Autodesk Fusion 360 part; units mm, degrees
(part 21 of 25)
  arc A482 (48.133, 42.8879) -> (48.133, 42.9641) centre (48.133, 42.926) ccw
  arc A483 (48.26, 36.9951) -> (48.26, 36.9189) centre (48.26, 36.957) ccw
  line L257 (48.895, 41.021) -> (48.895, 42.799)
  arc A484 (43.307, 39.1541) -> (43.307, 39.0779) centre (43.307, 39.116) ccw
  line L258 (48.133, 40.894) -> (43.307, 40.894)
  arc A485 (43.2801, 39.0891) -> (43.3339, 39.1429) centre (43.307, 39.116) ccw
  arc A486 (43.2069, 39.2699) -> (43.1531, 39.2161) centre (43.18, 39.243) ccw
  arc A487 (48.641, 36.9189) -> (48.641, 36.9951) centre (48.641, 36.957) ccw
  arc A488 (48.133, 37.0459) -> (48.133, 37.1221) centre (48.133, 37.084) ccw
  arc A489 (48.9331, 41.021) -> (48.8569, 41.021) centre (48.895, 41.021) ccw
  line L259 (42.799, 43.053) -> (43.18, 43.053)
  arc A490 (48.2869, 43.0261) -> (48.2331, 43.0799) centre (48.26, 43.053) ccw
  arc A491 (48.641, 43.0149) -> (48.641, 43.0911) centre (48.641, 43.053) ccw
  arc A492 (28.5369, 41.021) -> (28.6131, 41.021) centre (28.575, 41.021) ccw
  line L260 (42.799, 40.767) -> (43.18, 40.767)
  line L261 (48.133, 42.926) -> (43.307, 42.926)
  arc A493 (48.26, 40.8051) -> (48.26, 40.7289) centre (48.26, 40.767) ccw
  arc A494 (48.641, 40.8051) -> (48.641, 40.7289) centre (48.641, 40.767) ccw
  arc A495 (48.1061, 42.9529) -> (48.1599, 42.8991) centre (48.133, 42.926) ccw
  arc A496 (48.641, 43.0911) -> (48.641, 43.0149) centre (48.641, 43.053) ccw
  arc A497 (42.5831, 42.799) -> (42.5069, 42.799) centre (42.545, 42.799) ccw
  arc A498 (42.799, 40.8051) -> (42.799, 40.7289) centre (42.799, 40.767) ccw
  arc A499 (43.307, 42.9641) -> (43.307, 42.8879) centre (43.307, 42.926) ccw
  arc A500 (43.18, 43.0149) -> (43.18, 43.0911) centre (43.18, 43.053) ccw
  arc A501 (48.133, 40.8559) -> (48.133, 40.9321) centre (48.133, 40.894) ccw
  arc A502 (48.26, 43.0911) -> (48.26, 43.0149) centre (48.26, 43.053) ccw
  line L262 (29.337, 42.926) -> (29.21, 43.053)
  line L263 (48.641, 43.053) -> (48.26, 43.053)
  arc A503 (29.3639, 40.8671) -> (29.3101, 40.9209) centre (29.337, 40.894) ccw
  arc A504 (43.3339, 40.8671) -> (43.2801, 40.9209) centre (43.307, 40.894) ccw
  arc A505 (29.1831, 40.7939) -> (29.2369, 40.7401) centre (29.21, 40.767) ccw
  arc A506 (34.29, 43.0911) -> (34.29, 43.0149) centre (34.29, 43.053) ccw
  arc A507 (28.829, 40.8051) -> (28.829, 40.7289) centre (28.829, 40.767) ccw
  arc A508 (42.799, 43.0911) -> (42.799, 43.0149) centre (42.799, 43.053) ccw
  arc A509 (48.2331, 40.7401) -> (48.2869, 40.7939) centre (48.26, 40.767) ccw
  line L264 (34.163, 40.894) -> (34.29, 40.767)
  arc A510 (42.799, 43.053) -> (42.545, 42.799) centre (42.799, 42.799) ccw
  arc A511 (42.5069, 41.021) -> (42.5831, 41.021) centre (42.545, 41.021) ccw
  arc A512 (42.799, 43.0149) -> (42.799, 43.0911) centre (42.799, 43.053) ccw
  line L265 (42.545, 41.6052) -> (42.545, 42.2148)
  line L266 (49.7586, 41.6052) -> (49.7586, 42.2148)
  line L267 (41.6814, 42.2148) -> (41.6814, 41.6052)
  arc A513 (43.2069, 43.0799) -> (43.1531, 43.0261) centre (43.18, 43.053) ccw
  line L268 (28.829, 43.053) -> (29.21, 43.053)
  arc A514 (29.3101, 42.8991) -> (29.3639, 42.9529) centre (29.337, 42.926) ccw
  arc A515 (43.1531, 40.7939) -> (43.2069, 40.7401) centre (43.18, 40.767) ccw
  arc A516 (34.671, 40.7289) -> (34.671, 40.8051) centre (34.671, 40.767) ccw
  line L269 (43.307, 42.926) -> (43.18, 43.053)
  line L270 (34.671, 40.767) -> (34.29, 40.767)
  arc A517 (48.9331, 42.799) -> (48.8569, 42.799) centre (48.895, 42.799) ccw
  arc A518 (42.545, 41.021) -> (42.799, 40.767) centre (42.799, 41.021) ccw
  arc A519 (34.163, 42.8879) -> (34.163, 42.9641) centre (34.163, 42.926) ccw
  arc A520 (34.671, 40.767) -> (34.925, 41.021) centre (34.671, 41.021) ccw
  line L271 (28.575, 41.021) -> (28.575, 42.799)
  arc A521 (48.8569, 41.021) -> (48.9331, 41.021) centre (48.895, 41.021) ccw
  arc A522 (48.641, 40.7289) -> (48.641, 40.8051) centre (48.641, 40.767) ccw
  arc A523 (34.163, 40.8559) -> (34.163, 40.9321) centre (34.163, 40.894) ccw
  line L272 (48.133, 40.894) -> (48.26, 40.767)
  line L273 (42.545, 42.2148) -> (41.6814, 42.2148)
  line L274 (49.7586, 42.2148) -> (48.895, 42.2148)
  arc A524 (34.9631, 41.021) -> (34.8869, 41.021) centre (34.925, 41.021) ccw
  arc A525 (34.671, 43.0149) -> (34.671, 43.0911) centre (34.671, 43.053) ccw
  arc A526 (42.5831, 41.021) -> (42.5069, 41.021) centre (42.545, 41.021) ccw
  arc A527 (34.8869, 42.799) -> (34.9631, 42.799) centre (34.925, 42.799) ccw
  arc A528 (28.575, 41.021) -> (28.829, 40.767) centre (28.829, 41.021) ccw
  arc A529 (48.641, 40.767) -> (48.895, 41.021) centre (48.641, 41.021) ccw
  line L275 (41.6814, 41.6052) -> (42.545, 41.6052)
  arc A530 (34.671, 43.0911) -> (34.671, 43.0149) centre (34.671, 43.053) ccw
  arc A531 (13.081, 16.4211) -> (13.081, 16.3449) centre (13.081, 16.383) ccw
  arc A532 (28.6131, 42.799) -> (28.5369, 42.799) centre (28.575, 42.799) ccw
  arc A533 (34.9631, 42.799) -> (34.8869, 42.799) centre (34.925, 42.799) ccw
  arc A534 (13.081, 16.3449) -> (13.081, 16.4211) centre (13.081, 16.383) ccw
  arc A535 (34.925, 42.799) -> (34.671, 43.053) centre (34.671, 42.799) ccw
  arc A536 (34.29, 40.8051) -> (34.29, 40.7289) centre (34.29, 40.767) ccw
  arc A537 (28.829, 43.053) -> (28.575, 42.799) centre (28.829, 42.799) ccw
  arc A538 (29.337, 42.9641) -> (29.337, 42.8879) centre (29.337, 42.926) ccw
  arc A539 (34.2631, 40.7401) -> (34.3169, 40.7939) centre (34.29, 40.767) ccw
  arc A540 (29.21, 43.0149) -> (29.21, 43.0911) centre (29.21, 43.053) ccw
  arc A541 (34.671, 40.8051) -> (34.671, 40.7289) centre (34.671, 40.767) ccw
  arc A542 (28.829, 43.0149) -> (28.829, 43.0911) centre (28.829, 43.053) ccw
  arc A543 (7.7739, 14.1971) -> (7.7201, 14.2509) centre (7.747, 14.224) ccw
  line L276 (13.081, 16.383) -> (12.7, 16.383)
  line L277 (28.829, 40.767) -> (29.21, 40.767)
  line L278 (27.7114, 42.2148) -> (27.7114, 41.6052)
  arc A544 (28.6131, 41.021) -> (28.5369, 41.021) centre (28.575, 41.021) ccw
  line L279 (34.925, 41.021) -> (34.925, 42.799)
  arc A545 (34.3169, 43.0261) -> (34.2631, 43.0799) centre (34.29, 43.053) ccw
  arc A546 (12.5999, 14.2509) -> (12.5461, 14.1971) centre (12.573, 14.224) ccw
  arc A547 (7.6469, 16.4099) -> (7.5931, 16.3561) centre (7.62, 16.383) ccw
  arc A548 (29.21, 40.7289) -> (29.21, 40.8051) centre (29.21, 40.767) ccw
  line L280 (34.925, 41.6052) -> (35.7886, 41.6052)
  arc A549 (12.573, 14.1859) -> (12.573, 14.2621) centre (12.573, 14.224) ccw
  line L281 (28.575, 41.6052) -> (28.575, 42.2148)
  line L282 (35.7886, 42.2148) -> (34.925, 42.2148)
  arc A550 (28.829, 43.0911) -> (28.829, 43.0149) centre (28.829, 43.053) ccw
  line L283 (27.7114, 41.6052) -> (28.575, 41.6052)
  arc A551 (13.081, 14.097) -> (13.335, 14.351) centre (13.081, 14.351) ccw
  line L284 (7.747, 16.256) -> (12.573, 16.256)
  arc A552 (7.239, 16.383) -> (6.985, 16.129) centre (7.239, 16.129) ccw
  arc A553 (12.7, 14.1351) -> (12.7, 14.0589) centre (12.7, 14.097) ccw
  line L285 (12.573, 16.256) -> (12.7, 16.383)
  line L286 (13.335, 16.129) -> (13.335, 14.351)
  line L287 (29.337, 40.894) -> (29.21, 40.767)
  arc A554 (34.1899, 40.9209) -> (34.1361, 40.8671) centre (34.163, 40.894) ccw
  arc A555 (28.829, 40.7289) -> (28.829, 40.8051) centre (28.829, 40.767) ccw
  arc A556 (13.2969, 14.351) -> (13.3731, 14.351) centre (13.335, 14.351) ccw
  line L288 (35.7886, 41.6052) -> (35.7886, 42.2148)
  line L289 (34.671, 43.053) -> (34.29, 43.053)
  arc A557 (6.9469, 16.129) -> (7.0231, 16.129) centre (6.985, 16.129) ccw
  arc A558 (12.573, 16.2179) -> (12.573, 16.2941) centre (12.573, 16.256) ccw
  arc A559 (7.0231, 14.351) -> (6.9469, 14.351) centre (6.985, 14.351) ccw
  arc A560 (29.2369, 43.0799) -> (29.1831, 43.0261) centre (29.21, 43.053) ccw
  line L290 (13.081, 14.097) -> (12.7, 14.097)
  arc A561 (7.747, 16.2941) -> (7.747, 16.2179) centre (7.747, 16.256) ccw
  arc A562 (7.239, 14.0589) -> (7.239, 14.1351) centre (7.239, 14.097) ccw
  arc A563 (34.8869, 41.021) -> (34.9631, 41.021) centre (34.925, 41.021) ccw
  line L291 (7.747, 14.224) -> (7.62, 14.097)
  line L292 (34.925, 42.2148) -> (34.925, 41.6052)
  arc A564 (13.335, 16.129) -> (13.081, 16.383) centre (13.081, 16.129) ccw
  arc A565 (28.5369, 42.799) -> (28.6131, 42.799) centre (28.575, 42.799) ccw
  line L293 (34.163, 42.926) -> (34.29, 43.053)
  line L294 (12.573, 14.224) -> (12.7, 14.097)
  line L295 (34.163, 40.894) -> (29.337, 40.894)
  arc A566 (12.6731, 14.0701) -> (12.7269, 14.1239) centre (12.7, 14.097) ccw
  line L296 (34.163, 42.926) -> (29.337, 42.926)
  line L297 (28.575, 42.2148) -> (27.7114, 42.2148)
  line L298 (7.747, 16.256) -> (7.62, 16.383)
  arc A567 (29.337, 40.9321) -> (29.337, 40.8559) centre (29.337, 40.894) ccw
  arc A568 (34.1361, 42.9529) -> (34.1899, 42.8991) centre (34.163, 42.926) ccw
  arc A569 (13.3731, 16.129) -> (13.2969, 16.129) centre (13.335, 16.129) ccw
  arc A570 (13.081, 14.1351) -> (13.081, 14.0589) centre (13.081, 14.097) ccw
  arc A571 (12.7, 16.4211) -> (12.7, 16.3449) centre (12.7, 16.383) ccw
  line L299 (6.985, 15.5448) -> (6.1214, 15.5448)
  line L300 (7.747, 14.224) -> (12.573, 14.224)
  arc A572 (12.5461, 16.2829) -> (12.5999, 16.2291) centre (12.573, 16.256) ccw
  arc A573 (13.3731, 14.351) -> (13.2969, 14.351) centre (13.335, 14.351) ccw
  arc A574 (7.239, 16.3449) -> (7.239, 16.4211) centre (7.239, 16.383) ccw
  arc A575 (7.239, 14.1351) -> (7.239, 14.0589) centre (7.239, 14.097) ccw
  line L301 (6.1214, 14.9352) -> (6.985, 14.9352)
  arc A576 (7.62, 16.3449) -> (7.62, 16.4211) centre (7.62, 16.383) ccw
  arc A577 (7.62, 14.0589) -> (7.62, 14.1351) centre (7.62, 14.097) ccw
  arc A578 (12.7269, 16.3561) -> (12.6731, 16.4099) centre (12.7, 16.383) ccw
  arc A579 (7.747, 14.2621) -> (7.747, 14.1859) centre (7.747, 14.224) ccw
  arc A580 (6.9469, 14.351) -> (7.0231, 14.351) centre (6.985, 14.351) ccw
  arc A581 (13.2969, 16.129) -> (13.3731, 16.129) centre (13.335, 16.129) ccw
  arc A582 (13.081, 14.0589) -> (13.081, 14.1351) centre (13.081, 14.097) ccw
  arc A583 (6.985, 14.351) -> (7.239, 14.097) centre (7.239, 14.351) ccw
  line L302 (7.239, 14.097) -> (7.62, 14.097)
  arc A584 (7.5931, 14.1239) -> (7.6469, 14.0701) centre (7.62, 14.097) ccw
  arc A585 (7.7201, 16.2291) -> (7.7739, 16.2829) centre (7.747, 16.256) ccw
  line L303 (13.335, 14.9352) -> (14.1986, 14.9352)
  arc A586 (21.4559, 38.2265) -> (21.971, 38.545) centre (20.3211, 40.6376) ccw
  arc A587 (19.1706, 38.1983) -> (19.1976, 38.2557) centre (19.1841, 38.227) ccw
  arc A588 (80.4672, 18.034) -> (80.5688, 18.034) centre (80.518, 18.034) ccw
  arc A589 (5.207, 29.1465) -> (5.207, 29.2735) centre (5.207, 29.21) ccw
  arc A590 (80.5688, 20.048) -> (80.4672, 20.048) centre (80.518, 20.048) ccw
  line L304 (74.4499, 6.1715) -> (74.4499, 4.1275)
  arc A591 (7.62, 26.67) -> (7.62, 24.13) centre (7.62, 25.4) ccw
  arc A592 (4.5085, 28.575) -> (4.6355, 28.575) centre (4.572, 28.575) ccw
  arc A593 (7.239, 16.4211) -> (7.239, 16.3449) centre (7.239, 16.383) ccw
  arc A594 (80.4951, 4.1275) -> (80.5967, 4.1275) centre (80.5459, 4.1275) ccw
  arc A595 (74.3991, 4.1275) -> (74.5007, 4.1275) centre (74.4499, 4.1275) ccw
  line L305 (13.335, 15.5448) -> (13.335, 14.9352)
  arc A596 (75.311, 22.1488) -> (75.311, 22.0472) centre (75.311, 22.098) ccw
  arc A597 (7.62, 18.415) -> (7.62, 32.385) centre (7.62, 25.4) ccw
  line L306 (79.629, 22.098) -> (75.311, 22.098)
  arc A598 (79.629, 15.9512) -> (79.629, 16.0528) centre (79.629, 16.002) ccw
  line L307 (75.3389, 2.0955) -> (79.6569, 2.0955)
  line L308 (80.518, 20.048) -> (80.518, 18.034)
  arc A599 (4.6355, 29.845) -> (4.5085, 29.845) centre (4.572, 29.845) ccw
  line L309 (21.971, 38.545) -> (21.971, 42.735)
  line L310 (80.5459, 6.1415) -> (80.5459, 4.1275)
  arc A600 (79.6569, 8.1407) -> (79.6569, 8.2423) centre (79.6569, 8.1915) ccw
  arc A601 (75.3389, 2.1463) -> (75.3389, 2.0447) centre (75.3389, 2.0955) ccw
  arc A602 (77.47, 17.272) -> (77.47, 20.828) centre (77.47, 19.05) ccw
  arc A603 (77.47, 20.828) -> (77.47, 17.272) centre (77.47, 19.05) ccw
  line L311 (6.985, 14.9352) -> (6.985, 15.5448)
  arc A604 (77.4979, 6.9215) -> (77.4979, 3.3655) centre (77.4979, 5.1435) ccw
  arc A605 (4.572, 30.48) -> (4.572, 27.94) centre (4.572, 29.21) ccw
  arc A606 (7.62, 24.13) -> (7.62, 26.67) centre (7.62, 25.4) ccw
  arc A607 (77.4979, 3.3655) -> (77.4979, 6.9215) centre (77.4979, 5.1435) ccw
  arc A608 (75.311, 16.0528) -> (75.311, 15.9512) centre (75.311, 16.002) ccw
  line L312 (14.1986, 15.5448) -> (13.335, 15.5448)
  arc A609 (79.6569, 2.0447) -> (79.6569, 2.1463) centre (79.6569, 2.0955) ccw
  arc A610 (74.4728, 20.078) -> (74.3712, 20.078) centre (74.422, 20.078) ccw
  arc A611 (21.9513, 42.7101) -> (21.9907, 42.7599) centre (21.971, 42.735) ccw
  arc A612 (79.629, 22.0472) -> (79.629, 22.1488) centre (79.629, 22.098) ccw
  arc A613 (4.572, 27.94) -> (4.572, 30.48) centre (4.572, 29.21) ccw
  line L313 (4.572, 28.575) -> (4.572, 29.845)
  arc A614 (20.4788, 42.044) -> (20.4153, 42.044) centre (20.4471, 42.044) ccw
  line L314 (14.1986, 14.9352) -> (14.1986, 15.5448)
  line L315 (6.985, 16.129) -> (6.985, 14.351)
  arc A615 (75.3389, 8.2423) -> (75.3389, 8.1407) centre (75.3389, 8.1915) ccw
  arc A616 (7.0231, 16.129) -> (6.9469, 16.129) centre (6.985, 16.129) ccw
  line L316 (6.1214, 15.5448) -> (6.1214, 14.9352)
  line L317 (7.239, 16.383) -> (7.62, 16.383)
  arc A617 (80.5967, 6.1415) -> (80.4951, 6.1415) centre (80.5459, 6.1415) ccw
  line L318 (75.311, 16.002) -> (79.629, 16.002)
  arc A618 (74.3712, 18.034) -> (74.4728, 18.034) centre (74.422, 18.034) ccw
  line L319 (3.937, 29.21) -> (5.207, 29.21)
  arc A619 (7.62, 32.385) -> (7.62, 18.415) centre (7.62, 25.4) ccw
  arc A620 (3.937, 29.2735) -> (3.937, 29.1465) centre (3.937, 29.21) ccw
  arc A621 (74.5007, 6.1715) -> (74.3991, 6.1715) centre (74.4499, 6.1715) ccw
  line L320 (79.6569, 8.1915) -> (75.3389, 8.1915)
  line L321 (74.422, 20.078) -> (74.422, 18.034)
  arc A622 (21.445, 43.0936) -> (21.4186, 43.0358) centre (21.4318, 43.0647) ccw
  arc A623 (20.4788, 39.504) -> (20.4153, 39.504) centre (20.4471, 39.504) ccw
  arc A624 (20.4153, 39.236) -> (20.4788, 39.236) centre (20.4471, 39.236) ccw
  arc A625 (20.4153, 41.776) -> (20.4788, 41.776) centre (20.4471, 41.776) ccw
  arc A626 (22.0027, 42.735) -> (21.9393, 42.735) centre (21.971, 42.735) ccw
  line L322 (20.447, 42.044) -> (20.447, 41.776)
  arc A627 (21.9393, 38.545) -> (22.0027, 38.545) centre (21.971, 38.545) ccw
  arc A628 (19.1841, 43.053) -> (19.1841, 38.227) centre (20.3201, 40.64) ccw
  arc A629 (21.9907, 38.5201) -> (21.9513, 38.5699) centre (21.971, 38.545) ccw
  arc A630 (21.971, 42.735) -> (21.4318, 43.0647) centre (20.321, 40.6423) ccw
  arc A631 (21.4424, 38.2552) -> (21.4694, 38.1978) centre (21.4559, 38.2265) ccw
  arc A632 (19.1976, 43.0243) -> (19.1706, 43.0817) centre (19.1841, 43.053) ccw
  line L323 (20.447, 39.504) -> (20.447, 39.236)
  line L324 (75.311, 22.098) -> (74.422, 22.098)
  line L325 (74.422, 22.098) -> (74.422, 20.078)
  line L326 (74.422, 18.034) -> (74.422, 16.002)
  line L327 (74.422, 16.002) -> (75.311, 16.002)
  line L328 (79.629, 16.002) -> (80.518, 16.002)
  line L329 (80.518, 16.002) -> (80.518, 18.034)
  line L330 (79.629, 22.098) -> (80.518, 22.098)
  line L331 (80.518, 22.098) -> (80.518, 20.048)
  line L332 (75.3389, 8.1915) -> (74.4499, 8.1915)
  line L333 (74.4499, 8.1915) -> (74.4499, 6.1715)
  line L334 (74.4499, 4.1275) -> (74.4499, 2.0955)
  line L335 (74.4499, 2.0955) -> (75.3389, 2.0955)
  line L336 (79.6569, 2.0955) -> (80.5459, 2.0955)
  line L337 (80.5459, 2.0955) -> (80.5459, 4.1275)
  line L338 (79.6569, 8.1915) -> (80.5459, 8.1915)
  line L339 (80.5459, 8.1915) -> (80.5459, 6.1415)
  arc A633 (21.4318, 43.0647) -> (19.1841, 43.053) centre (20.3205, 40.6413) ccw
  arc A634 (19.1841, 38.227) -> (21.4559, 38.2265) centre (20.3205, 40.641) ccw
  arc A635 (14.8844, 6.2992) -> (13.0344, 6.283) centre (13.97, 5.0798) ccw
  arc A636 (13.0344, 3.877) -> (14.8558, 3.8399) centre (13.97, 5.0802) ccw
  arc A637 (5.9817, 6.2865) -> (4.1317, 6.2703) centre (5.0673, 5.0671) ccw
  arc A638 (4.1317, 3.8643) -> (5.9531, 3.8272) centre (5.0673, 5.0675) ccw
  constraint coincident A596.centre L306.end
  constraint perpendicular L321 L324
  constraint coincident A610.centre L321.start
  constraint perpendicular L324 L325
  constraint coincident A618.centre L321.end
  constraint perpendicular L318 L326
  constraint coincident A608.centre L318.start
  constraint perpendicular L326 L327
  constraint coincident A598.centre L318.end
  constraint perpendicular L308 L328
  constraint coincident A588.centre L308.end
  constraint perpendicular L328 L329
  constraint coincident L306.start A612.centre
  constraint perpendicular L308 L330
  constraint coincident A590.centre L308.start
  constraint perpendicular L330 L331
  constraint coincident A615.centre L320.end
  constraint perpendicular L304 L332
  constraint coincident L304.start A621.centre
  constraint perpendicular L332 L333
  constraint coincident L304.end A595.centre
  constraint perpendicular L307 L334
  constraint coincident L307.start A601.centre
  constraint perpendicular L334 L335
  constraint coincident L307.end A609.centre
  constraint perpendicular L310 L336
  constraint coincident A594.centre L310.end
  constraint perpendicular L336 L337
  constraint coincident A600.centre L320.start
  constraint perpendicular L310 L338
  constraint coincident L310.start A617.centre
  constraint perpendicular L320 L339
  constraint coincident A622.centre A630.end
  constraint tangent A630 A633
  constraint tangent A628 A634
  constraint tangent A222 A635
  constraint tangent A238 A636
  constraint tangent A171 A638
  constraint tangent A242 A637
sketch "Through Holes" plane through (0, 0, 0) normal (0, 0, 1) x (1, 0, 0)
  line L0 (72.5558, 49.13) -> (72.2242, 49.13)
  line L1 (72.2242, 49.13) -> (71.99, 49.3642)
  line L2 (72.7901, 49.6958) -> (72.7901, 49.3642)
  line L3 (72.2242, 49.9301) -> (72.5558, 49.9301)
  line L4 (74.53, 49.6958) -> (74.7642, 49.9301)
  line L5 (71.99, 49.3642) -> (71.99, 49.6958)
  arc A0 (68.1101, 6.35) -> (69.0499, 6.35) centre (68.58, 6.35) ccw
  line L6 (74.7642, 49.13) -> (74.53, 49.3642)
  line L7 (75.0958, 49.13) -> (74.7642, 49.13)
  line L8 (71.99, 49.6958) -> (72.2242, 49.9301)
  line L9 (74.7642, 49.9301) -> (75.0958, 49.9301)
  line L10 (72.2242, 49.9301) -> (72.5558, 49.9301)
  line L11 (74.53, 49.3642) -> (74.53, 49.6958)
  line L12 (75.0958, 49.13) -> (74.7642, 49.13)
  line L13 (75.3301, 49.3642) -> (75.0958, 49.13)
  line L14 (72.5558, 49.9301) -> (72.7901, 49.6958)
  arc A1 (66.5099, 6.35) -> (65.5701, 6.35) centre (66.04, 6.35) ccw
  line L15 (72.7901, 49.3642) -> (72.5558, 49.13)
  line L16 (74.7642, 49.9301) -> (75.0958, 49.9301)
  line L17 (74.7642, 49.13) -> (74.53, 49.3642)
  line L18 (72.7901, 49.3642) -> (72.5558, 49.13)
  line L19 (72.2242, 49.13) -> (71.99, 49.3642)
  line L20 (71.99, 49.3642) -> (71.99, 49.6958)
  line L21 (74.53, 49.6958) -> (74.7642, 49.9301)
  line L22 (71.99, 49.3642) -> (71.99, 49.6958)
  line L23 (75.3301, 49.3642) -> (75.0958, 49.13)
  line L24 (53.1558, 17.3355) -> (52.8955, 17.5958)
  line L25 (53.7845, 17.5958) -> (53.5242, 17.3355)
  arc A2 (50.8, 18.2245) -> (50.8, 17.3355) centre (50.8, 17.78) ccw
  line L26 (53.5242, 17.3355) -> (53.1558, 17.3355)
  line L27 (74.53, 49.3642) -> (74.53, 49.6958)
  arc A3 (50.8, 17.3355) -> (50.8, 18.2245) centre (50.8, 17.78) ccw
  line L28 (53.1558, 18.2245) -> (53.5242, 18.2245)
  arc A4 (50.8, 18.2245) -> (50.8, 17.3355) centre (50.8, 17.78) ccw
  line L29 (72.7901, 49.6958) -> (72.7901, 49.3642)
  line L30 (75.3301, 49.6958) -> (75.3301, 49.3642)
  line L31 (53.5242, 18.2245) -> (53.7845, 17.9642)
  line L32 (52.8955, 17.5958) -> (52.8955, 17.9642)
  line L33 (52.8955, 17.9642) -> (53.1558, 18.2245)
  arc A5 (65.5701, 6.35) -> (66.5099, 6.35) centre (66.04, 6.35) ccw
  line L34 (74.53, 49.3642) -> (74.53, 49.6958)
  arc A6 (69.0499, 6.35) -> (68.1101, 6.35) centre (68.58, 6.35) ccw
  line L35 (74.53, 49.3642) -> (74.53, 49.6958)
  line L36 (72.5558, 49.13) -> (72.2242, 49.13)
  line L37 (75.3301, 49.6958) -> (75.3301, 49.3642)
  line L38 (71.99, 49.6958) -> (72.2242, 49.9301)
  line L39 (72.5558, 49.9301) -> (72.7901, 49.6958)
  line L40 (52.8955, 17.5958) -> (52.8955, 17.9642)
  line L41 (75.0958, 49.9301) -> (75.3301, 49.6958)
  line L42 (75.0958, 49.9301) -> (75.3301, 49.6958)
  line L43 (71.99, 49.3642) -> (71.99, 49.6958)
  arc A7 (61.4299, 6.35) -> (60.4901, 6.35) centre (60.96, 6.35) ccw
  arc A8 (40.1701, 6.35) -> (41.1099, 6.35) centre (40.64, 6.35) ccw
  arc A9 (57.9501, 6.35) -> (58.8899, 6.35) centre (58.42, 6.35) ccw
  arc A10 (14.3891, 33.909) -> (13.5509, 33.909) centre (13.97, 33.909) ccw
  arc A11 (4.318, 50.3555) -> (4.318, 53.5305) centre (4.318, 51.943) ccw
  arc A12 (14.3891, 44.069) -> (13.5509, 44.069) centre (13.97, 44.069) ccw
  arc A13 (50.8, 17.3355) -> (50.8, 18.2245) centre (50.8, 17.78) ccw
  arc A14 (33.4899, 6.35) -> (32.5501, 6.35) centre (33.02, 6.35) ccw
  arc A15 (50.3301, 6.35) -> (51.2699, 6.35) centre (50.8, 6.35) ccw
  arc A16 (41.1099, 6.35) -> (40.1701, 6.35) centre (40.64, 6.35) ccw
  arc A17 (45.2501, 6.35) -> (46.1899, 6.35) centre (45.72, 6.35) ccw
  arc A18 (61.4299, 6.35) -> (60.4901, 6.35) centre (60.96, 6.35) ccw
  arc A19 (4.318, 50.3555) -> (4.318, 53.5305) centre (4.318, 51.943) ccw
  arc A20 (45.2501, 6.35) -> (46.1899, 6.35) centre (45.72, 6.35) ccw
  arc A21 (40.1701, 6.35) -> (41.1099, 6.35) centre (40.64, 6.35) ccw
  arc A22 (63.9699, 6.35) -> (63.0301, 6.35) centre (63.5, 6.35) ccw
  arc A23 (66.5099, 6.35) -> (65.5701, 6.35) centre (66.04, 6.35) ccw
  arc A24 (13.5509, 33.909) -> (14.3891, 33.909) centre (13.97, 33.909) ccw
  arc A25 (14.3891, 44.069) -> (13.5509, 44.069) centre (13.97, 44.069) ccw
  arc A26 (80.645, 50.3555) -> (80.645, 53.5305) centre (80.645, 51.943) ccw
  arc A27 (58.8899, 6.35) -> (57.9501, 6.35) centre (58.42, 6.35) ccw
  arc A28 (68.1101, 6.35) -> (69.0499, 6.35) centre (68.58, 6.35) ccw
  arc A29 (37.6301, 6.35) -> (38.5699, 6.35) centre (38.1, 6.35) ccw
  arc A30 (35.0901, 6.35) -> (36.0299, 6.35) centre (35.56, 6.35) ccw
  line L44 (53.1558, 18.2245) -> (53.5242, 18.2245)
  arc A31 (14.3891, 33.909) -> (13.5509, 33.909) centre (13.97, 33.909) ccw
  arc A32 (13.5509, 44.069) -> (14.3891, 44.069) centre (13.97, 44.069) ccw
  arc A33 (32.5501, 6.35) -> (33.4899, 6.35) centre (33.02, 6.35) ccw
  arc A34 (50.3301, 6.35) -> (51.2699, 6.35) centre (50.8, 6.35) ccw
  line L45 (53.7845, 17.5958) -> (53.5242, 17.3355)
  arc A35 (38.5699, 6.35) -> (37.6301, 6.35) centre (38.1, 6.35) ccw
  arc A36 (4.318, 53.5305) -> (4.318, 50.3555) centre (4.318, 51.943) ccw
  arc A37 (43.6499, 6.35) -> (42.7101, 6.35) centre (43.18, 6.35) ccw
  arc A38 (60.4901, 6.35) -> (61.4299, 6.35) centre (60.96, 6.35) ccw
  arc A39 (56.3499, 6.35) -> (55.4101, 6.35) centre (55.88, 6.35) ccw
  arc A40 (69.0499, 6.35) -> (68.1101, 6.35) centre (68.58, 6.35) ccw
  line L46 (52.8955, 17.5958) -> (52.8955, 17.9642)
  arc A41 (13.5509, 33.909) -> (14.3891, 33.909) centre (13.97, 33.909) ccw
  arc A42 (47.7901, 6.35) -> (48.7299, 6.35) centre (48.26, 6.35) ccw
  line L47 (53.5242, 17.3355) -> (53.1558, 17.3355)
  arc A43 (65.5701, 6.35) -> (66.5099, 6.35) centre (66.04, 6.35) ccw
  arc A44 (42.7101, 6.35) -> (43.6499, 6.35) centre (43.18, 6.35) ccw
  arc A45 (63.0301, 6.35) -> (63.9699, 6.35) centre (63.5, 6.35) ccw
  arc A46 (80.645, 53.5305) -> (80.645, 50.3555) centre (80.645, 51.943) ccw
  line L48 (53.7845, 17.9642) -> (53.7845, 17.5958)
  arc A47 (42.7101, 6.35) -> (43.6499, 6.35) centre (43.18, 6.35) ccw
  arc A48 (38.5699, 6.35) -> (37.6301, 6.35) centre (38.1, 6.35) ccw
  arc A49 (56.3499, 6.35) -> (55.4101, 6.35) centre (55.88, 6.35) ccw
  line L49 (52.8955, 17.5958) -> (52.8955, 17.9642)
  arc A50 (4.318, 53.5305) -> (4.318, 50.3555) centre (4.318, 51.943) ccw
  arc A51 (80.645, 50.3555) -> (80.645, 53.5305) centre (80.645, 51.943) ccw
  arc A52 (48.7299, 6.35) -> (47.7901, 6.35) centre (48.26, 6.35) ccw
  arc A53 (33.4899, 6.35) -> (32.5501, 6.35) centre (33.02, 6.35) ccw
  line L50 (52.8955, 17.9642) -> (53.1558, 18.2245)
  arc A54 (36.0299, 6.35) -> (35.0901, 6.35) centre (35.56, 6.35) ccw
  line L51 (53.1558, 17.3355) -> (52.8955, 17.5958)
  arc A55 (32.5501, 6.35) -> (33.4899, 6.35) centre (33.02, 6.35) ccw
  arc A56 (13.5509, 44.069) -> (14.3891, 44.069) centre (13.97, 44.069) ccw
  arc A57 (51.2699, 6.35) -> (50.3301, 6.35) centre (50.8, 6.35) ccw
  arc A58 (43.6499, 6.35) -> (42.7101, 6.35) centre (43.18, 6.35) ccw
  arc A59 (37.6301, 6.35) -> (38.5699, 6.35) centre (38.1, 6.35) ccw
  line L52 (53.5242, 18.2245) -> (53.7845, 17.9642)
  line L53 (53.7845, 17.9642) -> (53.7845, 17.5958)
  arc A60 (80.645, 53.5305) -> (80.645, 50.3555) centre (80.645, 51.943) ccw
  line L54 (40.7768, 32.6898) -> (40.5032, 32.6898)
  line L55 (50.4698, 32.8832) -> (50.4698, 33.1568)
  line L56 (40.3098, 32.8832) -> (40.3098, 33.1568)
  line L57 (40.9702, 32.8832) -> (40.7768, 32.6898)
  line L58 (51.1302, 33.1568) -> (51.1302, 32.8832)
  line L59 (40.9702, 32.8832) -> (40.7768, 32.6898)
  arc A61 (57.9501, 6.35) -> (58.8899, 6.35) centre (58.42, 6.35) ccw
  arc A62 (60.4901, 6.35) -> (61.4299, 6.35) centre (60.96, 6.35) ccw
  line L60 (51.1302, 32.8832) -> (50.9368, 32.6898)
  line L61 (50.6632, 32.6898) -> (50.4698, 32.8832)
  line L62 (40.5032, 32.6898) -> (40.3098, 32.8832)
  line L63 (50.4698, 33.1568) -> (50.6632, 33.3502)
  line L64 (50.6632, 33.3502) -> (50.9368, 33.3502)
  line L65 (50.9368, 33.3502) -> (51.1302, 33.1568)
  line L66 (51.1302, 33.1568) -> (51.1302, 32.8832)
  line L67 (40.3098, 33.1568) -> (40.5032, 33.3502)
  arc A63 (56.3499, 49.53) -> (55.4101, 49.53) centre (55.88, 49.53) ccw
  arc A64 (47.7901, 6.35) -> (48.7299, 6.35) centre (48.26, 6.35) ccw
  arc A65 (63.9699, 6.35) -> (63.0301, 6.35) centre (63.5, 6.35) ccw
  arc A66 (61.4299, 49.53) -> (60.4901, 49.53) centre (60.96, 49.53) ccw
  arc A67 (57.9501, 49.53) -> (58.8899, 49.53) centre (58.42, 49.53) ccw
  arc A68 (55.4101, 49.53) -> (56.3499, 49.53) centre (55.88, 49.53) ccw
  line L68 (40.9702, 33.1568) -> (40.9702, 32.8832)
  arc A69 (53.8099, 6.35) -> (52.8701, 6.35) centre (53.34, 6.35) ccw
  line L69 (40.5032, 32.6898) -> (40.3098, 32.8832)
  arc A70 (55.4101, 6.35) -> (56.3499, 6.35) centre (55.88, 6.35) ccw
  arc A71 (60.4901, 49.53) -> (61.4299, 49.53) centre (60.96, 49.53) ccw
  arc A72 (46.1899, 6.35) -> (45.2501, 6.35) centre (45.72, 6.35) ccw
  arc A73 (58.8899, 49.53) -> (57.9501, 49.53) centre (58.42, 49.53) ccw
  line L70 (50.9368, 32.6898) -> (50.6632, 32.6898)
  line L71 (40.9702, 33.1568) -> (40.9702, 32.8832)
  arc A74 (36.0299, 6.35) -> (35.0901, 6.35) centre (35.56, 6.35) ccw
  arc A75 (55.4101, 49.53) -> (56.3499, 49.53) centre (55.88, 49.53) ccw
  arc A76 (53.8099, 49.53) -> (52.8701, 49.53) centre (53.34, 49.53) ccw
  arc A77 (35.0901, 6.35) -> (36.0299, 6.35) centre (35.56, 6.35) ccw
  line L72 (40.5032, 33.3502) -> (40.7768, 33.3502)
  arc A78 (48.7299, 6.35) -> (47.7901, 6.35) centre (48.26, 6.35) ccw
  line L73 (50.6632, 32.6898) -> (50.4698, 32.8832)
  line L74 (40.3098, 32.8832) -> (40.3098, 33.1568)
  arc A79 (52.8701, 6.35) -> (53.8099, 6.35) centre (53.34, 6.35) ccw
  line L75 (50.4698, 33.1568) -> (50.6632, 33.3502)
  arc A80 (58.8899, 6.35) -> (57.9501, 6.35) centre (58.42, 6.35) ccw
  line L76 (40.5032, 33.3502) -> (40.7768, 33.3502)
  line L77 (40.3098, 33.1568) -> (40.5032, 33.3502)
  line L78 (40.9702, 33.1568) -> (40.9702, 32.8832)
  line L79 (40.7768, 33.3502) -> (40.9702, 33.1568)
  line L80 (40.7768, 33.3502) -> (40.9702, 33.1568)
  line L81 (40.7768, 32.6898) -> (40.5032, 32.6898)
  arc A81 (46.1899, 6.35) -> (45.2501, 6.35) centre (45.72, 6.35) ccw
  line L82 (50.6632, 33.3502) -> (50.9368, 33.3502)
  arc A82 (55.4101, 6.35) -> (56.3499, 6.35) centre (55.88, 6.35) ccw
  arc A83 (41.1099, 6.35) -> (40.1701, 6.35) centre (40.64, 6.35) ccw
  arc A84 (52.8701, 6.35) -> (53.8099, 6.35) centre (53.34, 6.35) ccw
  line L83 (50.9368, 33.3502) -> (51.1302, 33.1568)
  line L84 (51.1302, 32.8832) -> (50.9368, 32.6898)
  arc A85 (53.8099, 6.35) -> (52.8701, 6.35) centre (53.34, 6.35) ccw
  line L85 (51.1302, 33.1568) -> (51.1302, 32.8832)
  line L86 (51.1302, 33.1568) -> (51.1302, 32.8832)
  line L87 (40.9702, 33.1568) -> (40.9702, 32.8832)
  arc A86 (51.2699, 6.35) -> (50.3301, 6.35) centre (50.8, 6.35) ccw
  arc A87 (63.0301, 6.35) -> (63.9699, 6.35) centre (63.5, 6.35) ccw
  line L88 (50.9368, 32.6898) -> (50.6632, 32.6898)
  line L89 (50.4698, 32.8832) -> (50.4698, 33.1568)
  arc A88 (42.7101, 49.53) -> (43.6499, 49.53) centre (43.18, 49.53) ccw
  arc A89 (24.9301, 49.53) -> (25.8699, 49.53) centre (25.4, 49.53) ccw
  arc A90 (28.7401, 24.4602) -> (29.6799, 24.4602) centre (29.21, 24.4602) ccw
  arc A91 (51.2699, 49.53) -> (50.3301, 49.53) centre (50.8, 49.53) ccw
  arc A92 (33.8201, 24.4602) -> (34.7599, 24.4602) centre (34.29, 24.4602) ccw
  line L90 (29.21, 24.4602) -> (29.21, 26.3398)
  line L91 (36.83, 24.4602) -> (36.83, 26.3398)
  arc A93 (28.4099, 49.53) -> (27.4701, 49.53) centre (27.94, 49.53) ccw
  arc A94 (46.1899, 49.53) -> (45.2501, 49.53) centre (45.72, 49.53) ccw
  arc A95 (52.8701, 49.53) -> (53.8099, 49.53) centre (53.34, 49.53) ccw
  line L92 (34.29, 24.4602) -> (34.29, 26.3398)
  line L93 (31.75, 24.4602) -> (31.75, 26.3398)
  arc A96 (60.4901, 49.53) -> (61.4299, 49.53) centre (60.96, 49.53) ccw
  arc A97 (51.2699, 49.53) -> (50.3301, 49.53) centre (50.8, 49.53) ccw
  arc A98 (37.6301, 49.53) -> (38.5699, 49.53) centre (38.1, 49.53) ccw
  arc A99 (38.5699, 49.53) -> (37.6301, 49.53) centre (38.1, 49.53) ccw
  arc A100 (26.2001, 24.4602) -> (27.1399, 24.4602) centre (26.67, 24.4602) ccw
  arc A101 (30.9499, 49.53) -> (30.0101, 49.53) centre (30.48, 49.53) ccw
  arc A102 (24.9301, 49.53) -> (25.8699, 49.53) centre (25.4, 49.53) ccw
  arc A103 (48.7299, 49.53) -> (47.7901, 49.53) centre (48.26, 49.53) ccw
  arc A104 (32.5501, 49.53) -> (33.4899, 49.53) centre (33.02, 49.53) ccw
  arc A105 (25.8699, 49.53) -> (24.9301, 49.53) centre (25.4, 49.53) ccw
  arc A106 (37.6301, 49.53) -> (38.5699, 49.53) centre (38.1, 49.53) ccw
  arc A107 (30.0101, 49.53) -> (30.9499, 49.53) centre (30.48, 49.53) ccw
  arc A108 (45.2501, 49.53) -> (46.1899, 49.53) centre (45.72, 49.53) ccw
  arc A109 (43.6499, 49.53) -> (42.7101, 49.53) centre (43.18, 49.53) ccw
  arc A110 (41.1099, 49.53) -> (40.1701, 49.53) centre (40.64, 49.53) ccw
  arc A111 (50.3301, 49.53) -> (51.2699, 49.53) centre (50.8, 49.53) ccw
  arc A112 (48.7299, 49.53) -> (47.7901, 49.53) centre (48.26, 49.53) ccw
  arc A113 (57.9501, 49.53) -> (58.8899, 49.53) centre (58.42, 49.53) ccw
  arc A114 (25.8699, 49.53) -> (24.9301, 49.53) centre (25.4, 49.53) ccw
  arc A115 (43.6499, 49.53) -> (42.7101, 49.53) centre (43.18, 49.53) ccw
  arc A116 (47.7901, 49.53) -> (48.7299, 49.53) centre (48.26, 49.53) ccw
  arc A117 (56.3499, 49.53) -> (55.4101, 49.53) centre (55.88, 49.53) ccw
  arc A118 (28.4099, 49.53) -> (27.4701, 49.53) centre (27.94, 49.53) ccw
  arc A119 (27.4701, 49.53) -> (28.4099, 49.53) centre (27.94, 49.53) ccw
  arc A120 (46.1899, 49.53) -> (45.2501, 49.53) centre (45.72, 49.53) ccw
  arc A121 (32.5501, 49.53) -> (33.4899, 49.53) centre (33.02, 49.53) ccw
  arc A122 (45.2501, 49.53) -> (46.1899, 49.53) centre (45.72, 49.53) ccw
  arc A123 (33.4899, 49.53) -> (32.5501, 49.53) centre (33.02, 49.53) ccw
  arc A124 (61.4299, 49.53) -> (60.4901, 49.53) centre (60.96, 49.53) ccw
  arc A125 (30.9499, 49.53) -> (30.0101, 49.53) centre (30.48, 49.53) ccw
  arc A126 (42.7101, 49.53) -> (43.6499, 49.53) centre (43.18, 49.53) ccw
  arc A127 (40.1701, 49.53) -> (41.1099, 49.53) centre (40.64, 49.53) ccw
  arc A128 (30.0101, 49.53) -> (30.9499, 49.53) centre (30.48, 49.53) ccw
  arc A129 (38.5699, 49.53) -> (37.6301, 49.53) centre (38.1, 49.53) ccw
  arc A130 (35.0901, 49.53) -> (36.0299, 49.53) centre (35.56, 49.53) ccw
  arc A131 (41.1099, 49.53) -> (40.1701, 49.53) centre (40.64, 49.53) ccw
  line L94 (26.67, 24.4602) -> (26.67, 26.3398)
  arc A132 (58.8899, 49.53) -> (57.9501, 49.53) centre (58.42, 49.53) ccw
  arc A133 (33.4899, 49.53) -> (32.5501, 49.53) centre (33.02, 49.53) ccw
  arc A134 (53.8099, 49.53) -> (52.8701, 49.53) centre (53.34, 49.53) ccw
  arc A135 (36.0299, 49.53) -> (35.0901, 49.53) centre (35.56, 49.53) ccw
  arc A136 (28.7401, 24.4602) -> (29.6799, 24.4602) centre (29.21, 24.4602) ccw
  line L95 (29.21, 24.4602) -> (29.21, 26.3398)
  arc A137 (47.7901, 49.53) -> (48.7299, 49.53) centre (48.26, 49.53) ccw
  arc A138 (27.4701, 49.53) -> (28.4099, 49.53) centre (27.94, 49.53) ccw
  arc A139 (35.0901, 49.53) -> (36.0299, 49.53) centre (35.56, 49.53) ccw
  arc A140 (36.0299, 49.53) -> (35.0901, 49.53) centre (35.56, 49.53) ccw
  arc A141 (50.3301, 49.53) -> (51.2699, 49.53) centre (50.8, 49.53) ccw
  arc A142 (40.1701, 49.53) -> (41.1099, 49.53) centre (40.64, 49.53) ccw
  arc A143 (34.7599, 26.3398) -> (33.8201, 26.3398) centre (34.29, 26.3398) ccw
  arc A144 (52.8701, 49.53) -> (53.8099, 49.53) centre (53.34, 49.53) ccw
  arc A145 (27.1399, 26.3398) -> (26.2001, 26.3398) centre (26.67, 26.3398) ccw
  arc A146 (27.1399, 26.3398) -> (26.2001, 26.3398) centre (26.67, 26.3398) ccw
  arc A147 (36.3601, 24.4602) -> (37.2999, 24.4602) centre (36.83, 24.4602) ccw
  arc A148 (29.6799, 26.3398) -> (28.7401, 26.3398) centre (29.21, 26.3398) ccw
  line L96 (31.75, 24.4602) -> (31.75, 26.3398)
  arc A149 (37.2999, 26.3398) -> (36.3601, 26.3398) centre (36.83, 26.3398) ccw
  arc A150 (29.6799, 26.3398) -> (28.7401, 26.3398) centre (29.21, 26.3398) ccw
  arc A151 (31.2801, 24.4602) -> (32.2199, 24.4602) centre (31.75, 24.4602) ccw
  line L97 (34.29, 24.4602) -> (34.29, 26.3398)
  arc A152 (34.7599, 26.3398) -> (33.8201, 26.3398) centre (34.29, 26.3398) ccw
  arc A153 (26.2001, 24.4602) -> (27.1399, 24.4602) centre (26.67, 24.4602) ccw
  arc A154 (31.2801, 24.4602) -> (32.2199, 24.4602) centre (31.75, 24.4602) ccw
  line L98 (26.67, 24.4602) -> (26.67, 26.3398)
  arc A155 (32.2199, 26.3398) -> (31.2801, 26.3398) centre (31.75, 26.3398) ccw
  arc A156 (37.2999, 26.3398) -> (36.3601, 26.3398) centre (36.83, 26.3398) ccw
  arc A157 (74.1299, 32.6898) -> (73.1901, 32.6898) centre (73.66, 32.6898) ccw
  line L99 (78.74, 43.5102) -> (78.74, 45.3898)
  line L100 (76.2, 30.8102) -> (76.2, 32.6898)
  arc A158 (81.7499, 45.3898) -> (80.8101, 45.3898) centre (81.28, 45.3898) ccw
  arc A159 (79.2099, 45.3898) -> (78.2701, 45.3898) centre (78.74, 45.3898) ccw
  arc A160 (73.1901, 43.5102) -> (74.1299, 43.5102) centre (73.66, 43.5102) ccw
  line L101 (73.66, 43.5102) -> (73.66, 45.3898)
  line L102 (36.83, 24.4602) -> (36.83, 26.3398)
  line L103 (76.2, 43.5102) -> (76.2, 45.3898)
  arc A161 (81.7499, 45.3898) -> (80.8101, 45.3898) centre (81.28, 45.3898) ccw
  line L104 (78.74, 30.8102) -> (78.74, 32.6898)
  arc A162 (80.8101, 43.5102) -> (81.7499, 43.5102) centre (81.28, 43.5102) ccw
  arc A163 (73.1901, 30.8102) -> (74.1299, 30.8102) centre (73.66, 30.8102) ccw
  arc A164 (33.8201, 24.4602) -> (34.7599, 24.4602) centre (34.29, 24.4602) ccw
  arc A165 (79.2099, 45.3898) -> (78.2701, 45.3898) centre (78.74, 45.3898) ccw
  arc A166 (76.6699, 45.3898) -> (75.7301, 45.3898) centre (76.2, 45.3898) ccw
  arc A167 (76.6699, 45.3898) -> (75.7301, 45.3898) centre (76.2, 45.3898) ccw
  line L105 (73.66, 30.8102) -> (73.66, 32.6898)
  arc A168 (75.7301, 30.8102) -> (76.6699, 30.8102) centre (76.2, 30.8102) ccw
  line L106 (81.28, 43.5102) -> (81.28, 45.3898)
  line L107 (73.66, 30.8102) -> (73.66, 32.6898)
  arc A169 (74.1299, 45.3898) -> (73.1901, 45.3898) centre (73.66, 45.3898) ccw
  line L108 (73.66, 43.5102) -> (73.66, 45.3898)
  arc A170 (76.6699, 32.6898) -> (75.7301, 32.6898) centre (76.2, 32.6898) ccw
  arc A171 (75.7301, 30.8102) -> (76.6699, 30.8102) centre (76.2, 30.8102) ccw
  arc A172 (73.1901, 30.8102) -> (74.1299, 30.8102) centre (73.66, 30.8102) ccw
  arc A173 (78.2701, 43.5102) -> (79.2099, 43.5102) centre (78.74, 43.5102) ccw
  arc A174 (76.6699, 32.6898) -> (75.7301, 32.6898) centre (76.2, 32.6898) ccw
  arc A175 (74.1299, 45.3898) -> (73.1901, 45.3898) centre (73.66, 45.3898) ccw
  arc A176 (75.7301, 43.5102) -> (76.6699, 43.5102) centre (76.2, 43.5102) ccw
  arc A177 (75.7301, 43.5102) -> (76.6699, 43.5102) centre (76.2, 43.5102) ccw
  line L109 (76.2, 30.8102) -> (76.2, 32.6898)
  arc A178 (80.8101, 43.5102) -> (81.7499, 43.5102) centre (81.28, 43.5102) ccw
  arc A179 (36.3601, 24.4602) -> (37.2999, 24.4602) centre (36.83, 24.4602) ccw
  line L110 (81.28, 43.5102) -> (81.28, 45.3898)
  arc A180 (74.1299, 32.6898) -> (73.1901, 32.6898) centre (73.66, 32.6898) ccw
  arc A181 (78.2701, 43.5102) -> (79.2099, 43.5102) centre (78.74, 43.5102) ccw
  arc A182 (73.1901, 43.5102) -> (74.1299, 43.5102) centre (73.66, 43.5102) ccw
  arc A183 (32.2199, 26.3398) -> (31.2801, 26.3398) centre (31.75, 26.3398) ccw
  line L111 (78.74, 43.5102) -> (78.74, 45.3898)
  line L112 (76.2, 43.5102) -> (76.2, 45.3898)
  line L113 (63.5, 42.2402) -> (63.5, 44.1198)
  arc A184 (58.8899, 44.1198) -> (57.9501, 44.1198) centre (58.42, 44.1198) ccw
  line L114 (27.0701, 37.9342) -> (26.8358, 37.7)
  arc A185 (65.5701, 42.2402) -> (66.5099, 42.2402) centre (66.04, 42.2402) ccw
  line L115 (34.4558, 37.7) -> (34.1242, 37.7)
  line L116 (26.5042, 37.7) -> (26.27, 37.9342)
  arc A186 (81.7499, 32.6898) -> (80.8101, 32.6898) centre (81.28, 32.6898) ccw
  line L117 (66.04, 42.2402) -> (66.04, 44.1198)
  line L118 (63.5, 42.2402) -> (63.5, 44.1198)
  arc A187 (60.4901, 42.2402) -> (61.4299, 42.2402) centre (60.96, 42.2402) ccw
  arc A188 (66.5099, 44.1198) -> (65.5701, 44.1198) centre (66.04, 44.1198) ccw
  line L119 (33.89, 37.9342) -> (33.89, 38.2658)
  line L120 (34.1242, 37.7) -> (33.89, 37.9342)
  line L121 (34.69, 38.2658) -> (34.69, 37.9342)
  line L122 (34.69, 37.9342) -> (34.4558, 37.7)
  line L123 (34.4558, 37.7) -> (34.1242, 37.7)
  line L124 (34.69, 38.2658) -> (34.69, 37.9342)
  line L125 (34.1242, 38.5001) -> (34.4558, 38.5001)
  arc A189 (63.9699, 44.1198) -> (63.0301, 44.1198) centre (63.5, 44.1198) ccw
  line L126 (81.28, 30.8102) -> (81.28, 32.6898)
  arc A190 (80.8101, 30.8102) -> (81.7499, 30.8102) centre (81.28, 30.8102) ccw
  arc A191 (65.5701, 42.2402) -> (66.5099, 42.2402) centre (66.04, 42.2402) ccw
  arc A192 (65.5701, 30.8102) -> (66.5099, 30.8102) centre (66.04, 30.8102) ccw
  arc A193 (61.4299, 32.6898) -> (60.4901, 32.6898) centre (60.96, 32.6898) ccw
  line L127 (66.04, 42.2402) -> (66.04, 44.1198)
  arc A194 (63.9699, 44.1198) -> (63.0301, 44.1198) centre (63.5, 44.1198) ccw
  arc A195 (63.0301, 42.2402) -> (63.9699, 42.2402) centre (63.5, 42.2402) ccw
  arc A196 (79.2099, 32.6898) -> (78.2701, 32.6898) centre (78.74, 32.6898) ccw
  line L128 (26.8358, 37.7) -> (26.5042, 37.7)
  arc A197 (81.7499, 32.6898) -> (80.8101, 32.6898) centre (81.28, 32.6898) ccw
  arc A198 (63.0301, 30.8102) -> (63.9699, 30.8102) centre (63.5, 30.8102) ccw
  line L129 (34.69, 38.2658) -> (34.69, 37.9342)
  line L130 (34.4558, 38.5001) -> (34.69, 38.2658)
  arc A199 (60.4901, 42.2402) -> (61.4299, 42.2402) centre (60.96, 42.2402) ccw
  arc A200 (63.0301, 30.8102) -> (63.9699, 30.8102) centre (63.5, 30.8102) ccw
  arc A201 (61.4299, 44.1198) -> (60.4901, 44.1198) centre (60.96, 44.1198) ccw
  arc A202 (79.2099, 32.6898) -> (78.2701, 32.6898) centre (78.74, 32.6898) ccw
  line L131 (26.5042, 38.5001) -> (26.8358, 38.5001)
  line L132 (60.96, 42.2402) -> (60.96, 44.1198)
  arc A203 (57.9501, 42.2402) -> (58.8899, 42.2402) centre (58.42, 42.2402) ccw
  arc A204 (61.4299, 44.1198) -> (60.4901, 44.1198) centre (60.96, 44.1198) ccw
  line L133 (33.89, 38.2658) -> (34.1242, 38.5001)
  arc A205 (58.8899, 44.1198) -> (57.9501, 44.1198) centre (58.42, 44.1198) ccw
  line L134 (58.42, 42.2402) -> (58.42, 44.1198)
  line L135 (26.27, 37.9342) -> (26.27, 38.2658)
  line L136 (33.89, 38.2658) -> (34.1242, 38.5001)
  line L137 (34.69, 37.9342) -> (34.4558, 37.7)
  line L138 (33.89, 37.9342) -> (33.89, 38.2658)
  line L139 (81.28, 30.8102) -> (81.28, 32.6898)
  line L140 (58.42, 42.2402) -> (58.42, 44.1198)
  line L141 (27.0701, 38.2658) -> (27.0701, 37.9342)
  line L142 (60.96, 42.2402) -> (60.96, 44.1198)
  arc A206 (80.8101, 30.8102) -> (81.7499, 30.8102) centre (81.28, 30.8102) ccw
  line L143 (26.8358, 37.7) -> (26.5042, 37.7)
  arc A207 (63.0301, 42.2402) -> (63.9699, 42.2402) centre (63.5, 42.2402) ccw
  line L144 (34.4558, 38.5001) -> (34.69, 38.2658)
  line L145 (34.1242, 38.5001) -> (34.4558, 38.5001)
  arc A208 (78.2701, 30.8102) -> (79.2099, 30.8102) centre (78.74, 30.8102) ccw
  line L146 (26.27, 38.2658) -> (26.5042, 38.5001)
  arc A209 (57.9501, 42.2402) -> (58.8899, 42.2402) centre (58.42, 42.2402) ccw
  line L147 (34.1242, 37.7) -> (33.89, 37.9342)
  arc A210 (78.2701, 30.8102) -> (79.2099, 30.8102) centre (78.74, 30.8102) ccw
  line L148 (78.74, 30.8102) -> (78.74, 32.6898)
  arc A211 (66.5099, 44.1198) -> (65.5701, 44.1198) centre (66.04, 44.1198) ccw
  line L149 (34.69, 38.2658) -> (34.69, 37.9342)
  arc A212 (16.9799, 50.4698) -> (16.0401, 50.4698) centre (16.51, 50.4698) ccw
  line L150 (26.5042, 38.5001) -> (26.8358, 38.5001)
  arc A213 (61.4299, 32.6898) -> (60.4901, 32.6898) centre (60.96, 32.6898) ccw
  arc A214 (11.8999, 50.4698) -> (10.9601, 50.4698) centre (11.43, 50.4698) ccw
  line L151 (26.27, 37.9342) -> (26.27, 38.2658)
  line L152 (26.8358, 38.5001) -> (27.0701, 38.2658)
  arc A215 (65.5701, 30.8102) -> (66.5099, 30.8102) centre (66.04, 30.8102) ccw
  line L153 (27.0701, 38.2658) -> (27.0701, 37.9342)
  line L154 (60.96, 32.6898) -> (60.96, 30.8102)
  arc A216 (66.5099, 32.6898) -> (65.5701, 32.6898) centre (66.04, 32.6898) ccw
  line L155 (63.5, 32.6898) -> (63.5, 30.8102)
  arc A217 (19.5199, 50.4698) -> (18.5801, 50.4698) centre (19.05, 50.4698) ccw
  arc A218 (66.5099, 32.6898) -> (65.5701, 32.6898) centre (66.04, 32.6898) ccw
  line L156 (16.51, 50.4698) -> (16.51, 48.5902)
  line L157 (21.59, 50.4698) -> (21.59, 48.5902)
  arc A219 (13.5001, 48.5902) -> (14.4399, 48.5902) centre (13.97, 48.5902) ccw
  arc A220 (60.4901, 30.8102) -> (61.4299, 30.8102) centre (60.96, 30.8102) ccw
  line L158 (11.43, 50.4698) -> (11.43, 48.5902)
  line L159 (19.05, 50.4698) -> (19.05, 48.5902)
  arc A221 (14.4399, 50.4698) -> (13.5001, 50.4698) centre (13.97, 50.4698) ccw
  arc A222 (11.8999, 50.4698) -> (10.9601, 50.4698) centre (11.43, 50.4698) ccw
  line L160 (27.0701, 37.9342) -> (26.8358, 37.7)
  line L161 (66.04, 32.6898) -> (66.04, 30.8102)
  line L162 (26.8358, 38.5001) -> (27.0701, 38.2658)
  line L163 (13.97, 50.4698) -> (13.97, 48.5902)
  arc A223 (60.4901, 30.8102) -> (61.4299, 30.8102) centre (60.96, 30.8102) ccw
  arc A224 (22.0599, 50.4698) -> (21.1201, 50.4698) centre (21.59, 50.4698) ccw
  arc A225 (18.5801, 48.5902) -> (19.5199, 48.5902) centre (19.05, 48.5902) ccw
  arc A226 (13.5001, 48.5902) -> (14.4399, 48.5902) centre (13.97, 48.5902) ccw
  line L164 (11.43, 50.4698) -> (11.43, 48.5902)
  line L165 (26.5042, 34.69) -> (26.8358, 34.69)
  line L166 (34.69, 34.4558) -> (34.69, 34.1242)
  line L167 (26.8358, 34.69) -> (27.0701, 34.4558)
  arc A227 (21.1201, 48.5902) -> (22.0599, 48.5902) centre (21.59, 48.5902) ccw
  line L168 (26.27, 38.2658) -> (26.5042, 38.5001)
  arc A228 (21.1201, 48.5902) -> (22.0599, 48.5902) centre (21.59, 48.5902) ccw
  line L169 (13.97, 50.4698) -> (13.97, 48.5902)
  line L170 (19.05, 50.4698) -> (19.05, 48.5902)
  line L171 (27.0701, 34.4558) -> (27.0701, 34.1242)
  line L172 (26.27, 34.1242) -> (26.27, 34.4558)
  arc A229 (63.9699, 32.6898) -> (63.0301, 32.6898) centre (63.5, 32.6898) ccw
  arc A230 (16.9799, 50.4698) -> (16.0401, 50.4698) centre (16.51, 50.4698) ccw
  line L173 (26.5042, 33.89) -> (26.27, 34.1242)
  line L174 (27.0701, 34.4558) -> (27.0701, 34.1242)
  line L175 (27.0701, 38.2658) -> (27.0701, 37.9342)
  arc A231 (16.0401, 48.5902) -> (16.9799, 48.5902) centre (16.51, 48.5902) ccw
  arc A232 (10.9601, 48.5902) -> (11.8999, 48.5902) centre (11.43, 48.5902) ccw
  arc A233 (14.4399, 50.4698) -> (13.5001, 50.4698) centre (13.97, 50.4698) ccw
  line L176 (34.4558, 33.89) -> (34.1242, 33.89)
  line L177 (21.59, 50.4698) -> (21.59, 48.5902)
  line L178 (27.0701, 38.2658) -> (27.0701, 37.9342)
  arc A234 (19.5199, 50.4698) -> (18.5801, 50.4698) centre (19.05, 50.4698) ccw
  line L179 (60.96, 32.6898) -> (60.96, 30.8102)
  arc A235 (63.9699, 32.6898) -> (63.0301, 32.6898) centre (63.5, 32.6898) ccw
  arc A236 (16.0401, 48.5902) -> (16.9799, 48.5902) centre (16.51, 48.5902) ccw
  line L180 (63.5, 32.6898) -> (63.5, 30.8102)
  line L181 (34.4558, 33.89) -> (34.1242, 33.89)
  line L182 (34.69, 34.1242) -> (34.4558, 33.89)
  line L183 (26.5042, 37.7) -> (26.27, 37.9342)
  arc A237 (22.0599, 50.4698) -> (21.1201, 50.4698) centre (21.59, 50.4698) ccw
  arc A238 (10.9601, 48.5902) -> (11.8999, 48.5902) centre (11.43, 48.5902) ccw
  line L184 (66.04, 32.6898) -> (66.04, 30.8102)
  line L185 (16.51, 50.4698) -> (16.51, 48.5902)
  arc A239 (18.5801, 48.5902) -> (19.5199, 48.5902) centre (19.05, 48.5902) ccw
  line L186 (26.5042, 33.89) -> (26.27, 34.1242)
  arc A240 (50.3301, 24.4602) -> (51.2699, 24.4602) centre (50.8, 24.4602) ccw
  line L187 (48.26, 24.4602) -> (48.26, 26.3398)
  arc A241 (25.8699, 16.51) -> (24.9301, 16.51) centre (25.4, 16.51) ccw
  line L188 (34.69, 34.4558) -> (34.69, 34.1242)
  arc A242 (30.9499, 16.51) -> (30.0101, 16.51) centre (30.48, 16.51) ccw
  line L189 (26.8358, 33.89) -> (26.5042, 33.89)
  line L190 (53.34, 24.4602) -> (53.34, 26.3398)
  line L191 (34.1242, 34.69) -> (34.4558, 34.69)
  line L192 (33.89, 34.1242) -> (33.89, 34.4558)
  arc A243 (36.0299, 16.51) -> (35.0901, 16.51) centre (35.56, 16.51) ccw
  arc A244 (27.4701, 16.51) -> (28.4099, 16.51) centre (27.94, 16.51) ccw
  arc A245 (23.3299, 16.51) -> (22.3901, 16.51) centre (22.86, 16.51) ccw
  arc A246 (30.0101, 16.51) -> (30.9499, 16.51) centre (30.48, 16.51) ccw
  line L193 (27.0701, 34.1242) -> (26.8358, 33.89)
  arc A247 (27.4701, 16.51) -> (28.4099, 16.51) centre (27.94, 16.51) ccw
  arc A248 (33.4899, 16.51) -> (32.5501, 16.51) centre (33.02, 16.51) ccw
  arc A249 (51.2699, 26.3398) -> (50.3301, 26.3398) centre (50.8, 26.3398) ccw
  arc A250 (22.3901, 16.51) -> (23.3299, 16.51) centre (22.86, 16.51) ccw
  arc A251 (51.2699, 26.3398) -> (50.3301, 26.3398) centre (50.8, 26.3398) ccw
  line L194 (48.26, 24.4602) -> (48.26, 26.3398)
  arc A252 (47.7901, 24.4602) -> (48.7299, 24.4602) centre (48.26, 24.4602) ccw
  arc A253 (47.7901, 24.4602) -> (48.7299, 24.4602) centre (48.26, 24.4602) ccw
  line L195 (34.69, 34.4558) -> (34.69, 34.1242)
  arc A254 (22.3901, 16.51) -> (23.3299, 16.51) centre (22.86, 16.51) ccw
  line L196 (26.8358, 34.69) -> (27.0701, 34.4558)
  arc A255 (24.9301, 16.51) -> (25.8699, 16.51) centre (25.4, 16.51) ccw
  line L197 (27.0701, 34.4558) -> (27.0701, 34.1242)
  arc A256 (52.8701, 24.4602) -> (53.8099, 24.4602) centre (53.34, 24.4602) ccw
  line L198 (34.1242, 33.89) -> (33.89, 34.1242)
  line L199 (33.89, 34.4558) -> (34.1242, 34.69)
  arc A257 (50.3301, 24.4602) -> (51.2699, 24.4602) centre (50.8, 24.4602) ccw
  arc A258 (48.7299, 26.3398) -> (47.7901, 26.3398) centre (48.26, 26.3398) ccw
  line L200 (50.8, 24.4602) -> (50.8, 26.3398)
  line L201 (26.27, 34.4558) -> (26.5042, 34.69)
  line L202 (53.34, 24.4602) -> (53.34, 26.3398)
  arc A259 (33.4899, 16.51) -> (32.5501, 16.51) centre (33.02, 16.51) ccw
  line L203 (50.8, 24.4602) -> (50.8, 26.3398)
  line L204 (26.8358, 33.89) -> (26.5042, 33.89)
  arc A260 (28.4099, 16.51) -> (27.4701, 16.51) centre (27.94, 16.51) ccw
  line L205 (34.4558, 34.69) -> (34.69, 34.4558)
  line L206 (34.1242, 34.69) -> (34.4558, 34.69)
  line L207 (34.69, 34.1242) -> (34.4558, 33.89)
  arc A261 (23.3299, 16.51) -> (22.3901, 16.51) centre (22.86, 16.51) ccw
  arc A262 (32.5501, 16.51) -> (33.4899, 16.51) centre (33.02, 16.51) ccw
  arc A263 (53.8099, 26.3398) -> (52.8701, 26.3398) centre (53.34, 26.3398) ccw
  line L208 (33.89, 34.1242) -> (33.89, 34.4558)
  line L209 (26.5042, 34.69) -> (26.8358, 34.69)
  line L210 (26.27, 34.1242) -> (26.27, 34.4558)
  arc A264 (48.7299, 26.3398) -> (47.7901, 26.3398) centre (48.26, 26.3398) ccw
  arc A265 (24.9301, 16.51) -> (25.8699, 16.51) centre (25.4, 16.51) ccw
  line L211 (27.0701, 34.4558) -> (27.0701, 34.1242)
  line L212 (34.1242, 33.89) -> (33.89, 34.1242)
  line L213 (34.4558, 34.69) -> (34.69, 34.4558)
  arc A266 (53.8099, 26.3398) -> (52.8701, 26.3398) centre (53.34, 26.3398) ccw
  arc A267 (28.4099, 16.51) -> (27.4701, 16.51) centre (27.94, 16.51) ccw
  arc A268 (52.8701, 24.4602) -> (53.8099, 24.4602) centre (53.34, 24.4602) ccw
  arc A269 (30.9499, 16.51) -> (30.0101, 16.51) centre (30.48, 16.51) ccw
  line L214 (26.27, 34.4558) -> (26.5042, 34.69)
  line L215 (34.69, 34.4558) -> (34.69, 34.1242)
  line L216 (27.0701, 34.1242) -> (26.8358, 33.89)
  line L217 (33.89, 34.4558) -> (34.1242, 34.69)
  arc A270 (25.8699, 16.51) -> (24.9301, 16.51) centre (25.4, 16.51) ccw
  arc A271 (30.0101, 16.51) -> (30.9499, 16.51) centre (30.48, 16.51) ccw
  arc A272 (7.4676, 34.6202) -> (7.4676, 33.9598) centre (7.4676, 34.29) ccw
  arc A273 (2.3876, 34.6202) -> (2.3876, 33.9598) centre (2.3876, 34.29) ccw
  line L218 (7.4676, 41.91) -> (8.7884, 41.91)
  arc A274 (35.0901, 16.51) -> (36.0299, 16.51) centre (35.56, 16.51) ccw
  line L219 (4.8936, 6.7564) -> (5.241, 6.7564)
  arc A275 (3.7084, 44.1198) -> (3.7084, 44.7802) centre (3.7084, 44.45) ccw
  line L220 (2.3876, 44.45) -> (3.7084, 44.45)
  arc A276 (40.1701, 16.51) -> (41.1099, 16.51) centre (40.64, 16.51) ccw
  arc A277 (35.0901, 16.51) -> (36.0299, 16.51) centre (35.56, 16.51) ccw
  arc A278 (3.7084, 33.9598) -> (3.7084, 34.6202) centre (3.7084, 34.29) ccw